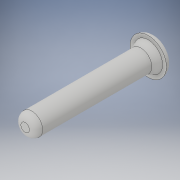
# Autodesk Inventor part: Globe_plug
Saved by Autodesk Inventor 2019.3 (Build 233278000, 278)
## iProperties
Created: 2020-09-27
Part Number: Globe_plug
Material: Generisch
Document SubType Name: Modeling
Designer: Nicolas Frick
Density: 1 g/cm^3
Appearance: Vorgabe
Author: Nicolas Frick
Autodesk Inventor part; units mm, degrees
ref_plane "YZ Plane" through (0, 0, 0) normal (1, 0, 0) x (0, 1, 0)
ref_plane "XZ Plane" through (0, 0, 0) normal (0, 1, 0) x (-1, 0, 0)
ref_plane "XY Plane" through (0, 0, 0) normal (0, 0, 1) x (1, 0, 0)
sketch "Skizze10" plane through (0, 0, 0) normal (1, 0, 0) x (0, 1, 0)
  line L0 (0, 0) -> (5.5, 0)
  line L1 (5.5, 0) -> (5.5, 2)
  line L2 (5.5, 2) -> (0, 2)
  line L3 (0, 2) -> (0, 0)
  line L4 (0, 2) -> (4.35, 2)
  line L5 (0, 2) -> (0, 4.2)
  line L6 (0, 4.2) -> (3.3, 4.2)
  line L7 (3.3, 4.2) -> (4.35, 2)
  line L8 (0, 4.2) -> (3.3, 4.2)
  line L9 (3.3, 4.2) -> (3.3, 39.2)
  line L10 (3.3, 39.2) -> (0, 39.2)
  line L11 (0, 39.2) -> (0, 4.2)
  dimension "d13" = 5.5
  dimension "d14" = 2
  dimension "d15" = 4.35
  dimension "d16" = 2.2
  dimension "d17" = 3.3
  dimension "d18" = 35
  constraints: 24 end point, 4 parallel, 3 horizontal, 2 perpendicular, 1 point on line, 1 vertical
  measures "d13" distance of L2.end L1.end
  measures "d14" distance of L1.end L0.end
  measures "d15" distance of L2.end L4.end
  measures "d16" distance of L2.end L5.end
  measures "d17" distance of L5.end L6.end
  measures "d18" distance of L9.end L8.end
revolve "Umdrehung1" add sketch "Skizze10" angle 360 about axis through (0, 0, 39.2) along (0, 0, -1)
fillet "Rundung1" radius 2 1 edges at (0, -5.5, 0)
fillet "Rundung2" radius 2 1 edges at (0, -3.3, 39.2)
